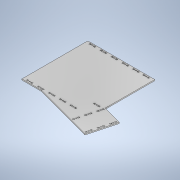
# Autodesk Inventor part: base_plate
Saved by Autodesk Inventor 2020.1 (Build 241239000, 239)
## iProperties
Created: 2019-07-16
Part Number: base_plate
Material: Générique
Document SubType Name: Modeling
Designer: Thibault
Density: 1 g/cm^3
Appearance: Aluminum - Poli
Author: Thibault
Autodesk Inventor part; units mm, degrees
ref_plane "YZ Plane" through (0, 0, 0) normal (1, 0, 0) x (0, 1, 0)
ref_plane "XZ Plane" through (0, 0, 0) normal (0, 1, 0) x (-1, 0, 0)
ref_plane "XY Plane" through (0, 0, 0) normal (0, 0, 1) x (1, 0, 0)
sketch "Anchor (screw side)" plane through (0, 0, 0) normal (0, 0, 1) x (1, 0, 0)
  circle A0 centre (93.7216, 50.3096) radius 1.05
  line L0 (91.2716, 51.3596) -> (88.1716, 51.3596)
  line L1 (88.1716, 51.3596) -> (88.1716, 49.2596)
  line L2 (88.1716, 49.2596) -> (91.2716, 49.2596)
  line L3 (91.2716, 49.2596) -> (91.2716, 51.3596)
  line L4 (99.2716, 51.3596) -> (96.1716, 51.3596)
  line L5 (96.1716, 51.3596) -> (96.1716, 49.2596)
  line L6 (96.1716, 49.2596) -> (99.2716, 49.2596)
  line L7 (99.2716, 49.2596) -> (99.2716, 51.3596)
  line L8 (91.2716, 51.3596) -> (96.1716, 49.2596) construction
  line L9 (96.1716, 51.3596) -> (91.2716, 49.2596) construction
  line L10 (86.1716, 53.3596) -> (101.2716, 53.3596) construction
  line L11 (101.2716, 53.3596) -> (101.2716, 47.2596) construction
  line L12 (101.2716, 47.2596) -> (86.1716, 47.2596) construction
  line L13 (86.1716, 47.2596) -> (86.1716, 53.3596) construction
  point P0 (103.5798, 50.1132)
  dimension "d27" = 2.1
  dimension "d28" = 3.1
  dimension "d29" = 2.1
  dimension "d32" = 4.9
  dimension "d34" = 2
  dimension "d35" = 2
  dimension "d36" = 2
  dimension "d37" = 2
  measures "d27" diameter of A0
  measures "d28" distance of L2.end L1.end
  measures "d29" distance of L1.end L0.end
  measures "d32" distance between parallel lines of L5 L3
  measures "d34" distance between parallel lines of L0 L10
  measures "d35" distance between parallel lines of L12 L2
  measures "d36" distance between parallel lines of L11 L7
  measures "d37" distance between parallel lines of L13 L1
sketch "Anchor (nut side)" plane through (0, 0, 0) normal (0, 0, 1) x (1, 0, 0)
  line L0 (10, 0) -> (8.55, 0)
  line L1 (8.55, 0) -> (8.55, -2)
  line L2 (8.55, -2) -> (9.35, -2)
  line L3 (9.35, -2) -> (9.35, -4)
  line L4 (5.65, -4) -> (5.65, -2)
  line L5 (5.65, -2) -> (6.45, -2)
  line L6 (6.45, -2) -> (6.45, 0)
  line L7 (6.45, 0) -> (5, 0)
  line L8 (2, 0) -> (2, 2)
  line L9 (2, 0) -> (3, 0) construction
  line L10 (2, 2) -> (5, 2)
  line L11 (5, 2) -> (5, 0)
  line L12 (10, 0) -> (10, 2)
  line L13 (10, 2) -> (13, 2)
  line L14 (13, 2) -> (13, 0)
  line L15 (0, 0) -> (2, 0)
  line L16 (13, 0) -> (15, 0)
  line L17 (5.65, -4) -> (6.45, -4)
  line L18 (9.35, -4) -> (8.55, -4)
  line L19 (6.45, -4) -> (6.45, -6.25)
  line L20 (8.55, -4) -> (8.55, -6.25)
  line L21 (6.7, -6.5) -> (7.5, -6.5)
  arc A0 (6.45, -6.25) -> (6.7, -6.5) centre (6.7, -6.25) ccw
  arc A1 (8.3, -6.5) -> (8.55, -6.25) centre (8.3, -6.25) ccw
  line L22 (7.5, -6.5) -> (8.3, -6.5)
  line L23 (7.5, -3.8983) -> (7.5, -9.959) construction
  point P0 (9.1321, -0.6227)
  point P1 (6.45, -6.5)
  point P2 (8.55, -6.5)
  dimension "d3" = 2
  dimension "d7" = 5
  dimension "d10" = 1.45
  dimension "d11" = 2
  dimension "d12" = 0.8
  dimension "d13" = 2
  dimension "d14" = 0.8
  dimension "d15" = 2.1
  dimension "d18" = 2
  dimension "d19" = 0.8
  dimension "d20" = 0.8
  dimension "d21" = 2.5
  dimension "d22" = 2.5
  dimension "d23" = 2.1
  dimension "d38" = 2
  dimension "d39" = 0.25
  dimension "d120" = 3
  measures "d3" distance of L15.start L8.start
  measures "d7" distance of L7.end L0.start
  measures "d10" distance of L0.start L0.end
  measures "d11" distance of L0.end L1.end
  measures "d12" distance of L1.end L2.end
  measures "d13" distance of L2.end L3.end
  measures "d14" distance of L4.end L5.end
  measures "d15" distance of L6.end L0.end
  measures "d18" distance of L14.end L16.end
  measures "d19" distance of L4.start L17.end
  measures "d20" distance of L3.end L18.end
  measures "d21" distance of L17.end point (6.45, -6.5)
  measures "d22" distance of L18.end point (8.55, -6.5)
  measures "d23" distance of L17.end L18.end
  measures "d38" distance between parallel lines of L15 L10
  measures "d39" radius of A0
  measures "d120" distance of L8.end L10.end
derived "shared_parameters.ipt"
sketch "Esquisse2" plane through (0, 0, 0) normal (0, 1, 0) x (-1, 0, 0)
  line L0 (-79.9773, 87.8545) -> (-182.0555, 87.8545)
  line L1 (-207.1187, 57.1167) -> (-207.1187, -37.2455)
  line L2 (-207.1187, -37.2455) -> (-81.9773, -37.2455)
  line L3 (-79.9773, -35.2455) -> (-79.9773, 87.8545)
  line L4 (-81.9773, -37.2455) -> (-79.9773, -35.2455)
  line L5 (-243.7891, 66.9425) -> (-230.0458, 118.2332)
  line L6 (-230.0458, 118.2332) -> (-191.3122, 107.8545)
  line L7 (-191.3122, 107.8545) -> (-205.0555, 56.5639)
  line L8 (-205.0555, 56.5639) -> (-243.7891, 66.9425)
  line L9 (-182.0555, 62.8129) -> (-203.3811, 62.8129)
  line L10 (-182.0555, 87.8545) -> (-182.0555, 62.8129)
  line L11 (-116.6712, 87.8545) -> (-191.3122, 107.8545)
  circle A0 centre (-91.7253, -34.1955) radius 1.05
  line L12 (-94.1753, -33.1455) -> (-97.2753, -33.1455)
  line L13 (-97.2753, -33.1455) -> (-97.2753, -35.2455)
  line L14 (-97.2753, -35.2455) -> (-94.1753, -35.2455)
  line L15 (-94.1753, -35.2455) -> (-94.1753, -33.1455)
  line L16 (-86.1753, -33.1455) -> (-89.2753, -33.1455)
  line L17 (-89.2753, -33.1455) -> (-89.2753, -35.2455)
  line L18 (-89.2753, -35.2455) -> (-86.1753, -35.2455)
  line L19 (-86.1753, -35.2455) -> (-86.1753, -33.1455)
  line L20 (-94.1753, -33.1455) -> (-89.2753, -35.2455) construction
  line L21 (-89.2753, -33.1455) -> (-94.1753, -35.2455) construction
  line L22 (-99.2753, -31.1455) -> (-84.1753, -31.1455) construction
  line L23 (-84.1753, -31.1455) -> (-84.1753, -37.2455) construction
  line L24 (-84.1753, -37.2455) -> (-99.2753, -37.2455) construction
  line L25 (-99.2753, -37.2455) -> (-99.2753, -31.1455) construction
  circle A1 centre (-112.7153, -34.1955) radius 1.05
  line L26 (-115.1653, -33.1455) -> (-118.2653, -33.1455)
  line L27 (-118.2653, -33.1455) -> (-118.2653, -35.2455)
  line L28 (-118.2653, -35.2455) -> (-115.1653, -35.2455)
  line L29 (-115.1653, -35.2455) -> (-115.1653, -33.1455)
  line L30 (-107.1653, -33.1455) -> (-110.2653, -33.1455)
  line L31 (-110.2653, -33.1455) -> (-110.2653, -35.2455)
  line L32 (-110.2653, -35.2455) -> (-107.1653, -35.2455)
  line L33 (-107.1653, -35.2455) -> (-107.1653, -33.1455)
  line L34 (-115.1653, -33.1455) -> (-110.2653, -35.2455) construction
  line L35 (-110.2653, -33.1455) -> (-115.1653, -35.2455) construction
  line L36 (-120.2653, -31.1455) -> (-105.1653, -31.1455) construction
  line L37 (-105.1653, -31.1455) -> (-105.1653, -37.2455) construction
  line L38 (-105.1653, -37.2455) -> (-120.2653, -37.2455) construction
  line L39 (-120.2653, -37.2455) -> (-120.2653, -31.1455) construction
  circle A2 centre (-133.6723, -34.1955) radius 1.05
  line L40 (-136.1223, -33.1455) -> (-139.2223, -33.1455)
  line L41 (-139.2223, -33.1455) -> (-139.2223, -35.2455)
  line L42 (-139.2223, -35.2455) -> (-136.1223, -35.2455)
  line L43 (-136.1223, -35.2455) -> (-136.1223, -33.1455)
  line L44 (-128.1223, -33.1455) -> (-131.2223, -33.1455)
  line L45 (-131.2223, -33.1455) -> (-131.2223, -35.2455)
  line L46 (-131.2223, -35.2455) -> (-128.1223, -35.2455)
  line L47 (-128.1223, -35.2455) -> (-128.1223, -33.1455)
  line L48 (-136.1223, -33.1455) -> (-131.2223, -35.2455) construction
  line L49 (-131.2223, -33.1455) -> (-136.1223, -35.2455) construction
  line L50 (-141.2223, -31.1455) -> (-126.1223, -31.1455) construction
  line L51 (-126.1223, -31.1455) -> (-126.1223, -37.2455) construction
  line L52 (-126.1223, -37.2455) -> (-141.2223, -37.2455) construction
  line L53 (-141.2223, -37.2455) -> (-141.2223, -31.1455) construction
  circle A3 centre (-154.3533, -34.1955) radius 1.05
  line L54 (-156.8033, -33.1455) -> (-159.9033, -33.1455)
  line L55 (-159.9033, -33.1455) -> (-159.9033, -35.2455)
  line L56 (-159.9033, -35.2455) -> (-156.8033, -35.2455)
  line L57 (-156.8033, -35.2455) -> (-156.8033, -33.1455)
  line L58 (-148.8033, -33.1455) -> (-151.9033, -33.1455)
  line L59 (-151.9033, -33.1455) -> (-151.9033, -35.2455)
  line L60 (-151.9033, -35.2455) -> (-148.8033, -35.2455)
  line L61 (-148.8033, -35.2455) -> (-148.8033, -33.1455)
  line L62 (-156.8033, -33.1455) -> (-151.9033, -35.2455) construction
  line L63 (-151.9033, -33.1455) -> (-156.8033, -35.2455) construction
  line L64 (-161.9033, -31.1455) -> (-146.8033, -31.1455) construction
  line L65 (-146.8033, -31.1455) -> (-146.8033, -37.2455) construction
  line L66 (-146.8033, -37.2455) -> (-161.9033, -37.2455) construction
  line L67 (-161.9033, -37.2455) -> (-161.9033, -31.1455) construction
  circle A4 centre (-174.5055, -34.1955) radius 1.05
  line L68 (-176.9555, -33.1455) -> (-180.0555, -33.1455)
  line L69 (-180.0555, -33.1455) -> (-180.0555, -35.2455)
  line L70 (-180.0555, -35.2455) -> (-176.9555, -35.2455)
  line L71 (-176.9555, -35.2455) -> (-176.9555, -33.1455)
  line L72 (-168.9555, -33.1455) -> (-172.0555, -33.1455)
  line L73 (-172.0555, -33.1455) -> (-172.0555, -35.2455)
  line L74 (-172.0555, -35.2455) -> (-168.9555, -35.2455)
  line L75 (-168.9555, -35.2455) -> (-168.9555, -33.1455)
  line L76 (-176.9555, -33.1455) -> (-172.0555, -35.2455) construction
  line L77 (-172.0555, -33.1455) -> (-176.9555, -35.2455) construction
  line L78 (-182.0555, -31.1455) -> (-166.9555, -31.1455) construction
  line L79 (-166.9555, -31.1455) -> (-166.9555, -37.2455) construction
  line L80 (-166.9555, -37.2455) -> (-182.0555, -37.2455) construction
  line L81 (-182.0555, -37.2455) -> (-182.0555, -31.1455) construction
  circle A5 centre (-193.8827, -34.1955) radius 1.05
  line L82 (-196.3327, -33.1455) -> (-199.4327, -33.1455)
  line L83 (-199.4327, -33.1455) -> (-199.4327, -35.2455)
  line L84 (-199.4327, -35.2455) -> (-196.3327, -35.2455)
  line L85 (-196.3327, -35.2455) -> (-196.3327, -33.1455)
  line L86 (-188.3327, -33.1455) -> (-191.4327, -33.1455)
  line L87 (-191.4327, -33.1455) -> (-191.4327, -35.2455)
  line L88 (-191.4327, -35.2455) -> (-188.3327, -35.2455)
  line L89 (-188.3327, -35.2455) -> (-188.3327, -33.1455)
  line L90 (-196.3327, -33.1455) -> (-191.4327, -35.2455) construction
  line L91 (-191.4327, -33.1455) -> (-196.3327, -35.2455) construction
  line L92 (-201.4327, -31.1455) -> (-186.3327, -31.1455) construction
  line L93 (-186.3327, -31.1455) -> (-186.3327, -37.2455) construction
  line L94 (-186.3327, -37.2455) -> (-201.4327, -37.2455) construction
  line L95 (-201.4327, -37.2455) -> (-201.4327, -31.1455) construction
  circle A6 centre (-91.7253, 84.8045) radius 1.05
  line L96 (-94.1753, 85.8545) -> (-97.2753, 85.8545)
  line L97 (-97.2753, 85.8545) -> (-97.2753, 83.7545)
  line L98 (-97.2753, 83.7545) -> (-94.1753, 83.7545)
  line L99 (-94.1753, 83.7545) -> (-94.1753, 85.8545)
  line L100 (-86.1753, 85.8545) -> (-89.2753, 85.8545)
  line L101 (-89.2753, 85.8545) -> (-89.2753, 83.7545)
  line L102 (-89.2753, 83.7545) -> (-86.1753, 83.7545)
  line L103 (-86.1753, 83.7545) -> (-86.1753, 85.8545)
  line L104 (-94.1753, 85.8545) -> (-89.2753, 83.7545) construction
  line L105 (-89.2753, 85.8545) -> (-94.1753, 83.7545) construction
  line L106 (-99.2753, 87.8545) -> (-84.1753, 87.8545) construction
  line L107 (-84.1753, 87.8545) -> (-84.1753, 81.7545) construction
  line L108 (-84.1753, 81.7545) -> (-99.2753, 81.7545) construction
  line L109 (-99.2753, 81.7545) -> (-99.2753, 87.8545) construction
  circle A7 centre (-112.7153, 84.8045) radius 1.05
  line L110 (-115.1653, 85.8545) -> (-118.2653, 85.8545)
  line L111 (-118.2653, 85.8545) -> (-118.2653, 83.7545)
  line L112 (-118.2653, 83.7545) -> (-115.1653, 83.7545)
  line L113 (-115.1653, 83.7545) -> (-115.1653, 85.8545)
  line L114 (-107.1653, 85.8545) -> (-110.2653, 85.8545)
  line L115 (-110.2653, 85.8545) -> (-110.2653, 83.7545)
  line L116 (-110.2653, 83.7545) -> (-107.1653, 83.7545)
  line L117 (-107.1653, 83.7545) -> (-107.1653, 85.8545)
  line L118 (-115.1653, 85.8545) -> (-110.2653, 83.7545) construction
  line L119 (-110.2653, 85.8545) -> (-115.1653, 83.7545) construction
  line L120 (-120.2653, 87.8545) -> (-105.1653, 87.8545) construction
  line L121 (-105.1653, 87.8545) -> (-105.1653, 81.7545) construction
  line L122 (-105.1653, 81.7545) -> (-120.2653, 81.7545) construction
  line L123 (-120.2653, 81.7545) -> (-120.2653, 87.8545) construction
  circle A8 centre (-133.6723, 84.8045) radius 1.05
  line L124 (-136.1223, 85.8545) -> (-139.2223, 85.8545)
  line L125 (-139.2223, 85.8545) -> (-139.2223, 83.7545)
  line L126 (-139.2223, 83.7545) -> (-136.1223, 83.7545)
  line L127 (-136.1223, 83.7545) -> (-136.1223, 85.8545)
  line L128 (-128.1223, 85.8545) -> (-131.2223, 85.8545)
  line L129 (-131.2223, 85.8545) -> (-131.2223, 83.7545)
  line L130 (-131.2223, 83.7545) -> (-128.1223, 83.7545)
  line L131 (-128.1223, 83.7545) -> (-128.1223, 85.8545)
  line L132 (-136.1223, 85.8545) -> (-131.2223, 83.7545) construction
  line L133 (-131.2223, 85.8545) -> (-136.1223, 83.7545) construction
  line L134 (-141.2223, 87.8545) -> (-126.1223, 87.8545) construction
  line L135 (-126.1223, 87.8545) -> (-126.1223, 81.7545) construction
  line L136 (-126.1223, 81.7545) -> (-141.2223, 81.7545) construction
  line L137 (-141.2223, 81.7545) -> (-141.2223, 87.8545) construction
  circle A9 centre (-154.3533, 84.8045) radius 1.05
  line L138 (-156.8033, 85.8545) -> (-159.9033, 85.8545)
  line L139 (-159.9033, 85.8545) -> (-159.9033, 83.7545)
  line L140 (-159.9033, 83.7545) -> (-156.8033, 83.7545)
  line L141 (-156.8033, 83.7545) -> (-156.8033, 85.8545)
  line L142 (-148.8033, 85.8545) -> (-151.9033, 85.8545)
  line L143 (-151.9033, 85.8545) -> (-151.9033, 83.7545)
  line L144 (-151.9033, 83.7545) -> (-148.8033, 83.7545)
  line L145 (-148.8033, 83.7545) -> (-148.8033, 85.8545)
  line L146 (-156.8033, 85.8545) -> (-151.9033, 83.7545) construction
  line L147 (-151.9033, 85.8545) -> (-156.8033, 83.7545) construction
  line L148 (-161.9033, 87.8545) -> (-146.8033, 87.8545) construction
  line L149 (-146.8033, 87.8545) -> (-146.8033, 81.7545) construction
  line L150 (-146.8033, 81.7545) -> (-161.9033, 81.7545) construction
  line L151 (-161.9033, 81.7545) -> (-161.9033, 87.8545) construction
  circle A10 centre (-174.5055, 84.8045) radius 1.05
  line L152 (-176.9555, 85.8545) -> (-180.0555, 85.8545)
  line L153 (-180.0555, 85.8545) -> (-180.0555, 83.7545)
  line L154 (-180.0555, 83.7545) -> (-176.9555, 83.7545)
  line L155 (-176.9555, 83.7545) -> (-176.9555, 85.8545)
  line L156 (-168.9555, 85.8545) -> (-172.0555, 85.8545)
  line L157 (-172.0555, 85.8545) -> (-172.0555, 83.7545)
  line L158 (-172.0555, 83.7545) -> (-168.9555, 83.7545)
  line L159 (-168.9555, 83.7545) -> (-168.9555, 85.8545)
  line L160 (-176.9555, 85.8545) -> (-172.0555, 83.7545) construction
  line L161 (-172.0555, 85.8545) -> (-176.9555, 83.7545) construction
  line L162 (-182.0555, 87.8545) -> (-166.9555, 87.8545) construction
  line L163 (-166.9555, 87.8545) -> (-166.9555, 81.7545) construction
  line L164 (-166.9555, 81.7545) -> (-182.0555, 81.7545) construction
  line L165 (-182.0555, 81.7545) -> (-182.0555, 87.8545) construction
  circle A11 centre (-193.8827, 59.7629) radius 1.05
  line L166 (-196.3327, 60.8129) -> (-199.4327, 60.8129)
  line L167 (-199.4327, 60.8129) -> (-199.4327, 58.7129)
  line L168 (-199.4327, 58.7129) -> (-196.3327, 58.7129)
  line L169 (-196.3327, 58.7129) -> (-196.3327, 60.8129)
  line L170 (-188.3327, 60.8129) -> (-191.4327, 60.8129)
  line L171 (-191.4327, 60.8129) -> (-191.4327, 58.7129)
  line L172 (-191.4327, 58.7129) -> (-188.3327, 58.7129)
  line L173 (-188.3327, 58.7129) -> (-188.3327, 60.8129)
  line L174 (-196.3327, 60.8129) -> (-191.4327, 58.7129) construction
  line L175 (-191.4327, 60.8129) -> (-196.3327, 58.7129) construction
  line L176 (-201.4327, 62.8129) -> (-186.3327, 62.8129) construction
  line L177 (-186.3327, 62.8129) -> (-186.3327, 56.7129) construction
  line L178 (-186.3327, 56.7129) -> (-201.4327, 56.7129) construction
  line L179 (-201.4327, 56.7129) -> (-201.4327, 62.8129) construction
  circle A12 centre (-238.8889, 73.4458) radius 1.05
  line L180 (-237.2406, 75.5406) -> (-236.4383, 78.535)
  line L181 (-236.4383, 78.535) -> (-238.4667, 79.0785)
  line L182 (-238.4667, 79.0785) -> (-239.2691, 76.0841)
  line L183 (-239.2691, 76.0841) -> (-237.2406, 75.5406)
  line L184 (-239.3112, 67.8132) -> (-238.5088, 70.8076)
  line L185 (-238.5088, 70.8076) -> (-240.5373, 71.3511)
  line L186 (-240.5373, 71.3511) -> (-241.3396, 68.3567)
  line L187 (-241.3396, 68.3567) -> (-239.3112, 67.8132)
  line L188 (-237.2406, 75.5406) -> (-240.5373, 71.3511) construction
  line L189 (-238.5088, 70.8076) -> (-239.2691, 76.0841) construction
  line L190 (-233.9888, 79.9492) -> (-237.897, 65.3637) construction
  line L191 (-237.897, 65.3637) -> (-243.7891, 66.9425) construction
  line L192 (-243.7891, 66.9425) -> (-239.8809, 81.528) construction
  line L193 (-239.8809, 81.528) -> (-233.9888, 79.9492) construction
  circle A13 centre (-233.9714, 91.7984) radius 1.05
  line L194 (-232.3231, 93.8932) -> (-231.5207, 96.8876)
  line L195 (-231.5207, 96.8876) -> (-233.5492, 97.4311)
  line L196 (-233.5492, 97.4311) -> (-234.3515, 94.4367)
  line L197 (-234.3515, 94.4367) -> (-232.3231, 93.8932)
  line L198 (-234.3936, 86.1658) -> (-233.5913, 89.1601)
  line L199 (-233.5913, 89.1601) -> (-235.6197, 89.7037)
  line L200 (-235.6197, 89.7037) -> (-236.4221, 86.7093)
  line L201 (-236.4221, 86.7093) -> (-234.3936, 86.1658)
  line L202 (-232.3231, 93.8932) -> (-235.6197, 89.7037) construction
  line L203 (-233.5913, 89.1601) -> (-234.3515, 94.4367) construction
  line L204 (-229.0712, 98.3018) -> (-232.9794, 83.7163) construction
  line L205 (-232.9794, 83.7163) -> (-238.8715, 85.2951) construction
  line L206 (-238.8715, 85.2951) -> (-234.9634, 99.8806) construction
  line L207 (-234.9634, 99.8806) -> (-229.0712, 98.3018) construction
  circle A14 centre (-229.0538, 110.151) radius 1.05
  line L208 (-227.4055, 112.2458) -> (-226.6032, 115.2401)
  line L209 (-226.6032, 115.2401) -> (-228.6316, 115.7837)
  line L210 (-228.6316, 115.7837) -> (-229.4339, 112.7893)
  line L211 (-229.4339, 112.7893) -> (-227.4055, 112.2458)
  line L212 (-229.476, 104.5184) -> (-228.6737, 107.5127)
  line L213 (-228.6737, 107.5127) -> (-230.7022, 108.0563)
  line L214 (-230.7022, 108.0563) -> (-231.5045, 105.0619)
  line L215 (-231.5045, 105.0619) -> (-229.476, 104.5184)
  line L216 (-227.4055, 112.2458) -> (-230.7022, 108.0563) construction
  line L217 (-228.6737, 107.5127) -> (-229.4339, 112.7893) construction
  line L218 (-224.1537, 116.6544) -> (-228.0618, 102.0689) construction
  line L219 (-228.0618, 102.0689) -> (-233.954, 103.6477) construction
  line L220 (-233.954, 103.6477) -> (-230.0458, 118.2332) construction
  line L221 (-230.0458, 118.2332) -> (-224.1537, 116.6544) construction
  circle A15 centre (-206.0475, 64.646) radius 1.05
  line L222 (-204.3991, 66.7407) -> (-203.5968, 69.7351)
  line L223 (-203.5968, 69.7351) -> (-205.6252, 70.2786)
  line L224 (-205.6252, 70.2786) -> (-206.4276, 67.2843)
  line L225 (-206.4276, 67.2843) -> (-204.3991, 66.7407)
  line L226 (-206.4697, 59.0133) -> (-205.6674, 62.0077)
  line L227 (-205.6674, 62.0077) -> (-207.6958, 62.5512)
  line L228 (-207.6958, 62.5512) -> (-208.4981, 59.5569)
  line L229 (-208.4981, 59.5569) -> (-206.4697, 59.0133)
  line L230 (-204.3991, 66.7407) -> (-207.6958, 62.5512) construction
  line L231 (-205.6674, 62.0077) -> (-206.4276, 67.2843) construction
  line L232 (-201.1473, 71.1493) -> (-205.0555, 56.5639) construction
  line L233 (-205.0555, 56.5639) -> (-210.9476, 58.1426) construction
  line L234 (-210.9476, 58.1426) -> (-207.0395, 72.7281) construction
  line L235 (-207.0395, 72.7281) -> (-201.1473, 71.1493) construction
  circle A16 centre (-201.1299, 82.9986) radius 1.05
  line L236 (-199.4816, 85.0933) -> (-198.6792, 88.0877)
  line L237 (-198.6792, 88.0877) -> (-200.7077, 88.6312)
  line L238 (-200.7077, 88.6312) -> (-201.51, 85.6369)
  line L239 (-201.51, 85.6369) -> (-199.4816, 85.0933)
  line L240 (-201.5521, 77.3659) -> (-200.7498, 80.3603)
  line L241 (-200.7498, 80.3603) -> (-202.7782, 80.9038)
  line L242 (-202.7782, 80.9038) -> (-203.5806, 77.9095)
  line L243 (-203.5806, 77.9095) -> (-201.5521, 77.3659)
  line L244 (-199.4816, 85.0933) -> (-202.7782, 80.9038) construction
  line L245 (-200.7498, 80.3603) -> (-201.51, 85.6369) construction
  line L246 (-196.2297, 89.5019) -> (-200.1379, 74.9164) construction
  line L247 (-200.1379, 74.9164) -> (-206.0301, 76.4952) construction
  line L248 (-206.0301, 76.4952) -> (-202.1219, 91.0807) construction
  line L249 (-202.1219, 91.0807) -> (-196.2297, 89.5019) construction
  circle A17 centre (-196.2123, 101.3512) radius 1.05
  line L250 (-194.564, 103.4459) -> (-193.7617, 106.4403)
  line L251 (-193.7617, 106.4403) -> (-195.7901, 106.9838)
  line L252 (-195.7901, 106.9838) -> (-196.5925, 103.9894)
  line L253 (-196.5925, 103.9894) -> (-194.564, 103.4459)
  line L254 (-196.6346, 95.7185) -> (-195.8322, 98.7129)
  line L255 (-195.8322, 98.7129) -> (-197.8607, 99.2564)
  line L256 (-197.8607, 99.2564) -> (-198.663, 96.262)
  line L257 (-198.663, 96.262) -> (-196.6346, 95.7185)
  line L258 (-194.564, 103.4459) -> (-197.8607, 99.2564) construction
  line L259 (-195.8322, 98.7129) -> (-196.5925, 103.9894) construction
  line L260 (-191.3122, 107.8545) -> (-195.2204, 93.269) construction
  line L261 (-195.2204, 93.269) -> (-201.1125, 94.8478) construction
  line L262 (-201.1125, 94.8478) -> (-197.2043, 109.4333) construction
  line L263 (-197.2043, 109.4333) -> (-191.3122, 107.8545) construction
  point P0 (0, 0)
  point P1 (-79.9773, -37.2455)
  dimension "d5" = 20.99
  dimension "d6" = 20.9571
  dimension "d8" = 20.681
  dimension "d9" = 20.1522
  dimension "d16" = 19.3773
  dimension "d41" = 96.0584
  dimension "d42" = 19
  dimension "d43" = 19
  dimension "d44" = 34
  dimension "d49" = 121.1
  dimension "d17" = 13.236
  dimension "d24" = 11.748
  dimension "d33" = 2
  dimension "d40" = 2
  dimension "angle" = 105
  dimension "dist_b" = 20
  dimension "dist_a" = 23
  constraints: 24 end point, 13 horizontal, 5 point on line, 4 parallel, 2 perpendicular, 2 vertical, 1 collinear, 4 other
  measures "d33" distance of L2.end point (-79.977, -37.245)
  measures "d40" distance of L3.start point (-79.977, -37.245)
  measures "angle" angle of L8 L10
  measures "dist_b" vertical distance of L6.end L0.end
  measures "dist_a" distance from line of L10 L7.end
extrude "Extrusion2" add sketch "Esquisse2" along normal blind 2
equation "\"d5\" = kws_bp_anchor_dist6"
equation "\"d6\" = kws_bp_anchor_dist5"
equation "\"d8\" = kws_bp_anchor_dist4"
equation "\"d9\" = kws_bp_anchor_dist3"
equation "\"d16\" = kws_bp_anchor_dist2"
equation "\"d41\" = short_switchplate_depth + extra_slot_dim"
equation "\"d42\" = tc_anchor_dist"
equation "\"d43\" = tc_anchor_dist"
equation "\"d44\" = tc_plates_dist"
equation "\"d17\" = kws_bp_anchor_dist1"
equation "\"d24\" = kws_bp_anchor_dist7"
equation "\"d40\" = d33"
equation "\"d25\" = sheet_thickness"
equation "\"kws_bp_anchor_dist6\" = 20.989966"
equation "\"kws_bp_anchor_dist5\" = 20.957071"
equation "\"kws_bp_anchor_dist4\" = 20.680956"
equation "\"kws_bp_anchor_dist3\" = 20.152201"
equation "\"kws_bp_anchor_dist2\" = 19.377266"
equation "\"short_switchplate_depth\" = 95.958352"
equation "\"extra_slot_dim\" = 0.1"
equation "\"tc_anchor_dist\" = 19"
equation "\"tc_plates_dist\" = 34"
equation "\"kws_bp_anchor_dist1\" = 13.236"
equation "\"kws_bp_anchor_dist7\" = 11.748"
equation "\"sheet_thickness\" = 2"
